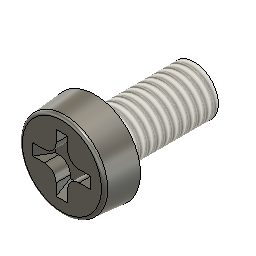
Stratus L1 Rocket (Autodesk Fusion 360 archive; units mm, degrees)
design "Cheese Head Screw ISO 7048 - M3 x 6 - H Steel 4.6 Plain"
description: Cheese Head Screw ISO 7048 - M3 x 6 - H
part number: ISO 7048 - H - M3 x 6 Steel 4.6 Plain
Autodesk Fusion 360 part; units mm, degrees
sketch "Sketch1" plane through (0, 0, 0) normal (0, 1, 0) x (1, 0, 0)
  line L0 (0, -2) -> (0, 6)
  line L1 (-2.75, 0) -> (-2.575, -2)
  line L2 (-2.75, 0) -> (-1.325, 0)
  line L3 (0, 6) -> (-1.5, 6)
  line L4 (-1.5, 6) -> (-1.5, 1)
  line L5 (-1.5, 1) -> (-1.325, 0.3469)
  line L6 (-1.325, 0.3469) -> (-1.325, 0)
  line L7 (0, -2) -> (-2.575, -2)
  dimension "d13" = 5
  dimension "d14" = 5.5
  dimension "d18" = 3
  dimension "d56" = 6
  dimension "d65" = 15
  dimension "d67" = 2
  dimension "d71" = 2.65
  dimension "d77" = 1
  constraint vertical L0
  constraint coincident origin L0
  constraint coincident origin L2
  constraint perpendicular L0 L3
  constraint coincident L2.end L6.end
  constraint perpendicular L0 L7
  measures "d13" angle of L0 L1
  measures "d56" distance of L2 L3
  measures "d65" angle of L5 L6
  measures "d67" distance of L1.start L7
  measures "d77" distance of L2 L4.end
revolve "Revolve1" add sketch "Sketch1" angle 360 about axis through (0, 0, 2) along (0, 0, -1) makes body 1
fillet "Fillet3" radius 0.2 1 edges at (-2.4008, 0.9312, 2) on bodies 1
fillet "Fillet2" radius 0.1 1 edges at (-1.2353, 0.4791, 0) on bodies 1
sketch "Sketch2" plane through (0, 0, 2) normal (0, 0, 1) x (1, 0, 0)
  line L0 (-0.35, 0.35) -> (-1.75, 0.35)
  line L1 (-1.75, 0.35) -> (-1.75, -0.35)
  line L2 (-1.75, -0.35) -> (-0.35, -0.35)
  line L3 (-0.35, -0.35) -> (-0.35, -1.75)
  line L4 (-0.35, -1.75) -> (0.35, -1.75)
  line L5 (0.35, -1.75) -> (0.35, -0.35)
  line L6 (0.35, -0.35) -> (1.75, -0.35)
  line L7 (1.75, -0.35) -> (1.75, 0.35)
  line L8 (1.75, 0.35) -> (0.35, 0.35)
  line L9 (0.35, 0.35) -> (0.35, 1.75)
  line L10 (0.35, 1.75) -> (-0.35, 1.75)
  line L11 (-0.35, 1.75) -> (-0.35, 0.35)
  dimension "d81" = 360
  dimension "d83" = 0.7
  dimension "d84" = 3.5
  constraint horizontal L0
  constraint perpendicular L0 L1
  constraint vertical L0.start L2.end
  constraint coincident L2.end L3.start
  measures "d83" distance of L0 L2
  measures "d84" distance of L1 L6.end
extrude "Extrude1" add sketch "Sketch2" against normal blind 0.86 separate body makes body 2
draft "Draft1" angle -30 neutral plane through (0, 0, 2) pull (0, 0, 1) 4 faces at (1.75, -0.1167, 1.7133) (0.1167, 1.75, 1.7133) (-1.75, 0.1167, 1.7133) (-0.1167, -1.75, 1.7133) on bodies 2
fillet "Fillet1" radius 0.7 4 edges at (-0.35, 0.35, 1.57) (-0.35, -0.35, 1.57) (0.35, -0.35, 1.57) (0.35, 0.35, 1.57) on bodies 2
combine "Combine1" operation cut target body 1 tool bodies 2
thread "Thread3" "ISO Metric profile 3.0 M3x0.5 M3x0.5 6g" major diameter 2.927 minor diameter 2.3555 pitch 0.5 angle 60 resizes the face on face at (-1.4981, -0.0748, -2.6667) on bodies 1
equation "adsk_nomdia = 3.00 mm"
equation "adsk_nomlen = 6.00 mm"
equation "adsk_headdia = 5.50 mm"
equation "adsk_phildia = 3.50 mm"
equation "adsk_midfillet = 0.10 mm"
equation "adsk_phildepth = 0.86 mm"
equation "adsk_shnklen = 1.00 mm"
equation "adsk_thrang = 15 deg"
equation "adsk_headang = 5 deg"
equation "d13 = adsk_headang"
equation "d14 = adsk_headdia"
equation "d18 = adsk_nomdia"
equation "adsk_philwidth = 0.70 mm"
equation "d43 = -adsk_phildepth"
equation "d52 = adsk_midfillet"
equation "d56 = adsk_nomlen"
equation "d65 = adsk_thrang"
equation "d67 = adsk_headh"
equation "adsk_headh = 2.00 mm"
equation "adsk_pitch1 = 0.50 mm"
equation "adsk_shnkdia = adsk_nomdia - 0.7 * adsk_pitch1"
equation "d71 = adsk_shnkdia"
equation "adsk_headtoprad = adsk_headh * 0.1"
equation "d76 = adsk_headtoprad"
equation "d77 = adsk_shnklen"
equation "d83 = adsk_philwidth"
equation "d84 = adsk_phildia"
equation "d86 = adsk_philwidth"

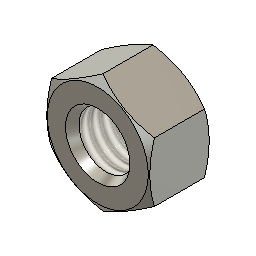
design "Hexagon Regular Nut ISO 4032 - M5 Steel 6 Plain"
description: Hexagon Regular Nut ISO 4032 - M5
part number: ISO 4032 - M5 Steel 6 Plain
Autodesk Fusion 360 part; units mm, degrees
sketch "Sketch1" plane through (0, 0, 0) normal (0, 1, 0) x (1, 0, 0)
  line L0 (0, 0) -> (0, -4.7)
  line L1 (-2.5, 0) -> (-3.92, 0)
  line L2 (-3.92, 0) -> (-4.62, -0.4041)
  line L3 (-4.62, -0.4041) -> (-4.62, -4.2959)
  line L4 (-4.62, -4.2959) -> (-3.92, -4.7)
  line L5 (-3.92, -4.7) -> (-2.5, -4.7)
  line L6 (-2.5, -4.7) -> (-2.5, 0)
  dimension "d121" = 5
  dimension "d122" = 30
  dimension "d123" = 30
  dimension "d128" = 9.24
  dimension "d172" = 7.84
  dimension "d179" = 4.7
  constraint vertical L0
  constraint coincident L0 L0.end
  constraint coincident origin L0
  constraint horizontal L1
  constraint coincident L0.start L1
  constraint coincident L0.start origin
  constraint coincident L0.end L5
  constraint vertical L1.end L4.end
  measures "d122" angle of L1 L2
  measures "d123" angle of L4 L5
  measures "d179" distance of L1 L5
revolve "Revolve1" add sketch "Sketch1" angle 360 about axis through (0, 0, 0) along (0, 0, 1)
sketch "Sketch8" plane through (0, 0, 4.7) normal (0, 0, 1) x (1, 0, 0)
  line L0 (-4, -2.3118) -> (-4, 2.3118)
  circle A0 centre (0, 0) radius 2.5
  circle A1 centre (0, 0) radius 4.62
  dimension "d114" = 4
  constraint coincident L0.end A1
  constraint coincident L0.start A1
  constraint vertical L0
  measures "d114" distance of A0.centre L0
extrude "Extrude5" cut sketch "Sketch8" against normal blind 4.7 contours L0 A1 picked at (-4.1, -0.5631)
pattern_circular "C-Pattern2" count 6 over 360 about axis through (0, 0, 1.75) along (0, 0, 1) of "Extrude5"
thread "Thread3" "ISO Metric profile 5.0 M5x0.8 M5x0.8 6H" major diameter 5.12 minor diameter 4.234 pitch 0.8 angle 60 resizes the face on face at (-2.4876, 0.2489, 3.1333)
sketch "Sketch12" plane through (0, 0, 0) normal (0, 1, 0) x (1, 0, 0)
  line L0 (-2.5, 0) -> (0, 0)
  line L1 (-1.1432, -2.35) -> (-2.5, 0)
  line L2 (-2.5, -4.7) -> (0, -4.7)
  line L3 (-1.1432, -2.35) -> (-2.5, -4.7)
  line L4 (0, 0) -> (0, -4.7)
  dimension "d169" = 60
  dimension "d177" = 2.5
  dimension "d178" = 60
  constraint horizontal L0
  constraint coincident L1.start L3.start
  constraint vertical L0.start L2.start
  constraint coincident L2.end L4.end
  constraint coincident L0.end L4.start
  constraint perpendicular L2 L4
  measures "d169" angle of L2 L3
  measures "d177" distance of L0.start L4
  measures "d178" angle of L0 L1
revolve "Revolve3" cut sketch "Sketch12" angle 360 about axis through (0, 0, 1.75) along (0, 0, 1)
equation "adsk_nheig = 4.70 mm"
equation "adsk_maxdia = 9.24 mm"
equation "adsk_nomdia = 5.00 mm"
equation "d89 = -adsk_nheig"
equation "adsk_waflat = 8.00 mm"
equation "d114 = adsk_waflat / 2"
equation "adsk_chamang1 = 30.00 deg"
equation "adsk_chamang2 = 30.00 deg"
equation "d121 = adsk_nomdia"
equation "d122 = adsk_chamang1"
equation "d123 = adsk_chamang2"
equation "d128 = adsk_maxdia"
equation "d163 = adsk_nheig"
equation "adsk_beardia = 7.84 mm"
equation "d172 = adsk_beardia"
equation "d177 = adsk_nomdia * 0.5"
equation "d179 = adsk_nheig"

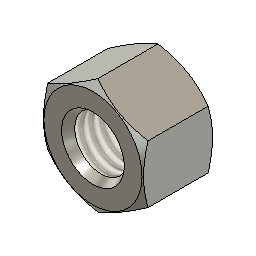
design "Hexagon Regular Nut ISO 4034 - M5 Steel 6 Plain"
description: Hexagon Regular Nut ISO 4034 - M5
part number: ISO 4034 - M5 Steel 6 Plain
Autodesk Fusion 360 part; units mm, degrees
sketch "Sketch1" plane through (0, 0, 0) normal (0, 1, 0) x (1, 0, 0)
  line L0 (0, 0) -> (0, -5.6)
  line L1 (-2.5, 0) -> (-3.92, 0)
  line L2 (-3.92, 0) -> (-4.62, -0.4041)
  line L3 (-4.62, -0.4041) -> (-4.62, -5.1959)
  line L4 (-4.62, -5.1959) -> (-3.92, -5.6)
  line L5 (-3.92, -5.6) -> (-2.5, -5.6)
  line L6 (-2.5, -5.6) -> (-2.5, 0)
  dimension "d121" = 5
  dimension "d122" = 30
  dimension "d123" = 30
  dimension "d128" = 9.24
  dimension "d172" = 7.84
  dimension "d179" = 5.6
  constraint vertical L0
  constraint coincident L0 L0.end
  constraint coincident origin L0
  constraint horizontal L1
  constraint coincident L0.start L1
  constraint coincident L0.start origin
  constraint coincident L0.end L5
  constraint vertical L1.end L4.end
  measures "d122" angle of L1 L2
  measures "d123" angle of L4 L5
  measures "d179" distance of L1 L5
revolve "Revolve1" add sketch "Sketch1" angle 360 about axis through (0, 0, 0) along (0, 0, 1)
sketch "Sketch8" plane through (0, 0, 5.6) normal (0, 0, 1) x (1, 0, 0)
  line L0 (-4, -2.3118) -> (-4, 2.3118)
  circle A0 centre (0, 0) radius 2.5
  circle A1 centre (0, 0) radius 4.62
  dimension "d114" = 4
  constraint coincident L0.end A1
  constraint coincident L0.start A1
  constraint vertical L0
  measures "d114" distance of A0.centre L0
extrude "Extrude5" cut sketch "Sketch8" against normal blind 5.6 contours L0 A1 picked at (-4.1, 0.5631)
pattern_circular "C-Pattern2" count 6 over 360 about axis through (0, 0, 1.75) along (0, 0, 1) of "Extrude5"
thread "Thread3" "ISO Metric profile 5.0 M5x0.8 M5x0.8 6H" major diameter 5.12 minor diameter 4.234 pitch 0.8 angle 60 resizes the face on face at (-2.4969, 0.1246, 3.7333)
sketch "Sketch12" plane through (0, 0, 0) normal (0, 1, 0) x (1, 0, 0)
  line L0 (-2.5, 0) -> (0, 0)
  line L1 (-0.8834, -2.8) -> (-2.5, 0)
  line L2 (-2.5, -5.6) -> (0, -5.6)
  line L3 (-0.8834, -2.8) -> (-2.5, -5.6)
  line L4 (0, 0) -> (0, -5.6)
  dimension "d169" = 60
  dimension "d177" = 2.5
  dimension "d178" = 60
  constraint horizontal L0
  constraint coincident L1.start L3.start
  constraint vertical L0.start L2.start
  constraint coincident L2.end L4.end
  constraint coincident L0.end L4.start
  constraint perpendicular L2 L4
  measures "d169" angle of L2 L3
  measures "d177" distance of L0.start L4
  measures "d178" angle of L0 L1
revolve "Revolve3" cut sketch "Sketch12" angle 360 about axis through (0, 0, 1.75) along (0, 0, 1)
equation "adsk_nheig = 5.60 mm"
equation "adsk_maxdia = 9.24 mm"
equation "adsk_nomdia = 5.00 mm"
equation "d89 = -adsk_nheig"
equation "adsk_waflat = 8.00 mm"
equation "d114 = adsk_waflat / 2"
equation "adsk_chamang1 = 30.00 deg"
equation "adsk_chamang2 = 30.00 deg"
equation "d121 = adsk_nomdia"
equation "d122 = adsk_chamang1"
equation "d123 = adsk_chamang2"
equation "d128 = adsk_maxdia"
equation "d163 = adsk_nheig"
equation "adsk_beardia = 7.84 mm"
equation "d172 = adsk_beardia"
equation "d177 = adsk_nomdia * 0.5"
equation "d179 = adsk_nheig"

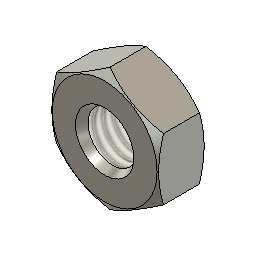
design "Hexagon Regular Nut ISO 4032 - M3 Steel 6 Plain"
description: Hexagon Regular Nut ISO 4032 - M3
part number: ISO 4032 - M3 Steel 6 Plain
Autodesk Fusion 360 part; units mm, degrees
sketch "Sketch1" plane through (0, 0, 0) normal (0, 1, 0) x (1, 0, 0)
  line L0 (0, 0) -> (0, -2.4)
  line L1 (-1.5, 0) -> (-2.695, 0)
  line L2 (-2.695, 0) -> (-3.1763, -0.2778)
  line L3 (-3.1763, -0.2778) -> (-3.1763, -2.1222)
  line L4 (-3.1763, -2.1222) -> (-2.695, -2.4)
  line L5 (-2.695, -2.4) -> (-1.5, -2.4)
  line L6 (-1.5, -2.4) -> (-1.5, 0)
  dimension "d121" = 3
  dimension "d122" = 30
  dimension "d123" = 30
  dimension "d128" = 6.3525
  dimension "d172" = 5.39
  dimension "d179" = 2.4
  constraint vertical L0
  constraint coincident L0 L0.end
  constraint coincident origin L0
  constraint horizontal L1
  constraint coincident L0.start L1
  constraint coincident L0.start origin
  constraint coincident L0.end L5
  constraint vertical L1.end L4.end
  measures "d122" angle of L1 L2
  measures "d123" angle of L4 L5
  measures "d179" distance of L1 L5
revolve "Revolve1" add sketch "Sketch1" angle 360 about axis through (0, 0, 0) along (0, 0, 1)
sketch "Sketch8" plane through (0, 0, 2.4) normal (0, 0, 1) x (1, 0, 0)
  line L0 (-2.75, -1.5894) -> (-2.75, 1.5894)
  circle A0 centre (0, 0) radius 1.5
  circle A1 centre (0, 0) radius 3.1763
  dimension "d114" = 2.75
  constraint coincident L0.end A1
  constraint coincident L0.start A1
  constraint vertical L0
  measures "d114" distance of A0.centre L0
extrude "Extrude5" cut sketch "Sketch8" against normal blind 2.4 contours L0 A1 picked at (-2.8188, -0.3871)
pattern_circular "C-Pattern2" count 6 over 360 about axis through (0, 0, 1.75) along (0, 0, 1) of "Extrude5"
thread "Thread3" "ISO Metric profile 3.0 M3x0.5 M3x0.5 6H" major diameter 3.086 minor diameter 2.529 pitch 0.5 angle 60 resizes the face on face at (-1.4925, 0.1494, 1.6)
sketch "Sketch12" plane through (0, 0, 0) normal (0, 1, 0) x (1, 0, 0)
  line L0 (-1.5, 0) -> (0, 0)
  line L1 (-0.8072, -1.2) -> (-1.5, 0)
  line L2 (-1.5, -2.4) -> (0, -2.4)
  line L3 (-0.8072, -1.2) -> (-1.5, -2.4)
  line L4 (0, 0) -> (0, -2.4)
  dimension "d169" = 60
  dimension "d177" = 1.5
  dimension "d178" = 60
  constraint horizontal L0
  constraint coincident L1.start L3.start
  constraint vertical L0.start L2.start
  constraint coincident L2.end L4.end
  constraint coincident L0.end L4.start
  constraint perpendicular L2 L4
  measures "d169" angle of L2 L3
  measures "d177" distance of L0.start L4
  measures "d178" angle of L0 L1
revolve "Revolve3" cut sketch "Sketch12" angle 360 about axis through (0, 0, 1.75) along (0, 0, 1)
equation "adsk_nheig = 2.40 mm"
equation "adsk_maxdia = 6.3525 mm"
equation "adsk_nomdia = 3.00 mm"
equation "d89 = -adsk_nheig"
equation "adsk_waflat = 5.50 mm"
equation "d114 = adsk_waflat / 2"
equation "adsk_chamang1 = 30.00 deg"
equation "adsk_chamang2 = 30.00 deg"
equation "d121 = adsk_nomdia"
equation "d122 = adsk_chamang1"
equation "d123 = adsk_chamang2"
equation "d128 = adsk_maxdia"
equation "d163 = adsk_nheig"
equation "adsk_beardia = 5.39 mm"
equation "d172 = adsk_beardia"
equation "d177 = adsk_nomdia * 0.5"
equation "d179 = adsk_nheig"
